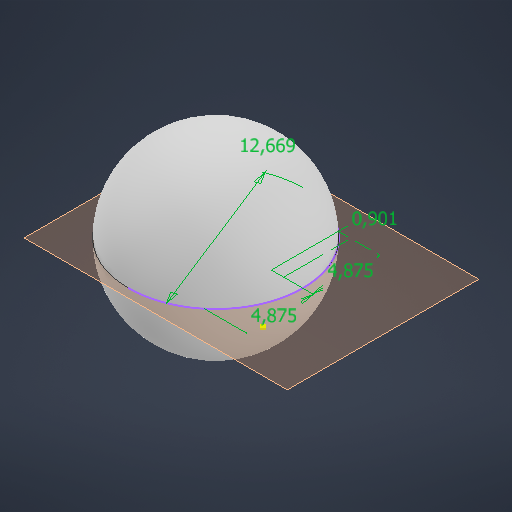
# Autodesk Inventor part: guscio sferico
Saved by Autodesk Inventor 2027 (Build 310192060, 192F)
## iProperties
Created: 2026-07-02
Part Number: guscio sferico
Material: Generic
Document SubType Name: Modeling
Designer: loren
Density: 1 g/cm^3
Appearance: Default
Author: loren
Autodesk Inventor part; units mm, degrees
ref_plane "YZ Plane" through (0, 0, 0) normal (1, 0, 0) x (0, 1, 0)
ref_plane "XY Plane" through (0, 0, 0) normal (0, 0, 1) x (1, 0, 0)
sketch "Sketch1" plane through (0, 0, 0) normal (0, 1, 0) x (-1, 0, 0)
  line L0 (33.043, -39.215) -> (33.043, 9.535)
  line L1 (33.043, -39.215) -> (33.043, -87.965)
  arc A0 (73.4942, 24.1322) -> (73.4942, -102.5622) centre (73.4942, -39.215) ccw
  line L2 (33.043, -39.215) -> (33.043, -87.965)
  line L3 (73.4942, 24.1322) -> (73.4942, -102.5622)
  point P0 (0, 0)
  point P1 (24.033, -39.215)
  dimension "d6" = 9.01
  dimension "d8" = 48.75
  dimension "d9" = 48.75
  dimension "d10" = 126.6944
  constraints: 8 end point, 3 point on circle, 2 vertical, 1 centre point, 1 collinear
  measures "d6" distance of L0.start point (24.033, -39.215)
  measures "d8" distance of L0.start L0.end
  measures "d9" distance of L0.start L1.end
  measures "d10" diameter of A0
revolve "Revolution1" add sketch "Sketch1" angle 360 about axis through (-73.4942, 0, 24.1322) along (0, 0, -1)
shell "Shell1" thickness 2 removed faces 0
split body "Split2" result two bodies by plane through (0, 0, 0) normal (0, 1, 0) first body at (-25.4319, 40.3291, -42.8692)
body "Solid2"
body "Solid3"
